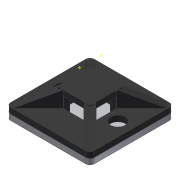
# Autodesk Inventor part: Klebesockel_HC-101SBK
Saved by Autodesk Inventor 2015 (Build 190159000, 159)
## iProperties
Created: 2015-01-25
Part Number: Klebesockel_HC-101SBK
Material: Generic
Document SubType Name: Modeling
Density: 1 g/cm^3
Appearance: Plastic_Black
Autodesk Inventor part; units mm, degrees
ref_plane "YZ Plane" through (0, 0, 0) normal (1, 0, 0) x (0, 1, 0)
sketch "Sketch1" plane through (0, 0, 0) normal (0, 0, 1) x (1, 0, 0)
  line L0 (-9.75, -9.75) -> (9.75, -9.75)
  line L1 (9.75, -9.75) -> (9.75, 9.75)
  line L2 (9.75, 9.75) -> (-9.75, 9.75)
  line L3 (-9.75, 9.75) -> (-9.75, -9.75)
  line L4 (-9.75, -9.75) -> (9.75, 9.75) construction
  line L5 (9.75, -9.75) -> (-9.75, 9.75) construction
  point P0 (0, 0)
  dimension "d0" = 19.5
  dimension "d1" = 19.5
  constraints: 12 end point, 2 midpoint, 2 parallel, 1 horizontal, 1 perpendicular
  measures "d0" distance of L2.end L1.end
  measures "d1" distance of L0.end L1.end
extrude "Extrusion1" add sketch "Sketch1" along normal blind 1.35
sketch "Sketch2" plane through (0, 0, 1.35) normal (0, 0, 1) x (1, 0, 0)
  line L0 (-3.8, -3.8) -> (3.8, -3.8)
  line L1 (3.8, -3.8) -> (3.8, 3.8)
  line L2 (3.8, 3.8) -> (-3.8, 3.8)
  line L3 (-3.8, 3.8) -> (-3.8, -3.8)
  line L4 (-3.8, -3.8) -> (3.8, 3.8) construction
  line L5 (3.8, -3.8) -> (-3.8, 3.8) construction
  point P0 (0, 0)
  dimension "d4" = 7.6
  dimension "d5" = 7.6
  constraints: 12 end point, 2 midpoint, 2 parallel, 1 horizontal, 1 perpendicular
  measures "d4" distance of L2.end L1.end
  measures "d5" distance of L0.end L1.end
extrude "Extrusion2" add sketch "Sketch2" along normal blind 3.7
fillet "Fillet1" radius 1 4 edges at (9.75, -9.75, 0.675) (9.75, 9.75, 0.675) (-9.75, -9.75, 0.675) (-9.75, 9.75, 0.675)
ref_plane "Work Plane1" through (0, 0, 0) normal (-0.7071, 0.7071, 0) x (0, 0, 1)
sketch "Sketch3" plane through (0, 0, 0) normal (-0.7071, 0.7071, 0) x (0, 0, 1)
  line L0 (5.05, 4.4) -> (1.35, 12.7)
  line L1 (1.35, 12.7) -> (1.35, 4.4)
  line L2 (1.35, 4.4) -> (5.05, 4.4)
  line L3 (1.35, 13.0815) -> (1.35, 0.7071) projected
  line L4 (5.05, 5.374) -> (5.05, 0) projected
  point P0 (0, 0)
  dimension "d10" = 4.4
  dimension "d11" = 12.7
  constraints: 6 end point, 1 collinear, 1 horizontal, 1 point on line, 1 vertical
  measures "d10" distance from line of point (0, 0) L2
  measures "d11" vertical distance of point (0, 0) L0.end
extrude "Extrusion3" add sketch "Sketch3" along normal mid plane 1.9
pattern_circular "Circular Pattern1" count 4 over 360 about axis through (0, 0, -10) along (0, 0, 1) of "Extrusion3"
sketch "Sketch4" plane through (0, 0, 0) normal (0, 0, -1) x (-1, 0, 0)
  line L0 (2.35, 3.8) -> (-2.35, 3.8)
  line L1 (-2.35, 3.8) -> (-2.35, -3.8)
  line L2 (-2.35, -3.8) -> (2.35, -3.8)
  line L3 (2.35, -3.8) -> (2.35, 3.8)
  line L4 (2.35, 3.8) -> (-2.35, -3.8) construction
  line L5 (-2.35, 3.8) -> (2.35, -3.8) construction
  line L6 (3.8, 2.35) -> (-3.8, 2.35)
  line L7 (-3.8, 2.35) -> (-3.8, -2.35)
  line L8 (-3.8, -2.35) -> (3.8, -2.35)
  line L9 (3.8, -2.35) -> (3.8, 2.35)
  line L10 (3.8, 2.35) -> (-3.8, -2.35) construction
  line L11 (-3.8, 2.35) -> (3.8, -2.35) construction
  line L12 (3.8, -3.8) -> (-3.8, -3.8) projected
  line L13 (-3.8, -3.8) -> (-3.8, 3.8) projected
  point P0 (0, 0)
  dimension "d17" = 4.7
  dimension "d18" = 4.7
  constraints: 24 end point, 4 midpoint, 4 parallel, 2 collinear, 2 horizontal, 2 perpendicular
  measures "d17" distance of L6.end L7.end
  measures "d18" distance of L1.end L2.end
extrude "Extrusion4" cut sketch "Sketch4" against normal blind 3.75 contours L3 L6 L1 L0 | L6 L9 L8 L3 | L3 L8 L1 L6 | L1 L8 L7 L6 | L3 L2 L1 L8
sketch "Sketch5" plane through (0, 0, 1.35) normal (0, 0, 1) x (1, 0, 0)
  point P0 (0, 0)
  point P1 (-6.5, 0)
  point P2 (6.5, 0)
  dimension "d22" = 13
  dimension "d23" = 6.5
  constraints: 2 horizontal alignment
  measures "d22" distance of point (6.5, 0) point (-6.5, 0)
  measures "d23" distance of point (0, 0) point (-6.5, 0)
hole "Hole1" at (-6.5, 0, 1.35) at (6.5, 0, 1.35) direction (0, 0, -1) diameter 3.4 end through all
sketch "Sketch6" plane through (0, 0, 0) normal (0, 0, -1) x (-1, 0, 0)
  line L0 (-8.75, 9.75) -> (8.75, 9.75) projected
  line L1 (-9.75, -8.75) -> (-9.75, 8.75) projected
  line L2 (8.75, -9.75) -> (-8.75, -9.75) projected
  line L3 (9.75, 8.75) -> (9.75, -8.75) projected
  arc A0 (8.75, -9.75) -> (9.75, -8.75) centre (8.75, -8.75) ccw projected
  arc A1 (-9.75, -8.75) -> (-8.75, -9.75) centre (-8.75, -8.75) ccw projected
  arc A2 (-8.75, 9.75) -> (-9.75, 8.75) centre (-8.75, 8.75) ccw projected
  arc A3 (9.75, 8.75) -> (8.75, 9.75) centre (8.75, 8.75) ccw projected
extrude "Extrusion5" add sketch "Sketch6" along normal blind 1.3 separate body
ref_plane "Work Plane2" through (0, 0, 10.05) normal (0, 0, 1) x (1, 0, 0)
sketch "Sketch7" plane through (0, 0, 10.05) normal (0, 0, 1) x (1, 0, 0)
  point P0 (0, 0)
  point P1 (0, -2.5)
  point P2 (0, 2.5)
  dimension "d34" = 5
  dimension "d35" = 2.5
  constraints: 2 vertical alignment
  measures "d34" distance of point (0, 2.5) point (0, -2.5)
  measures "d35" distance of point (0, 0) point (0, -2.5)
equation "\"d1\" = d0"
equation "\"d5\" = d4"
equation "\"d18\" = d17"
equation "\"d23\" = 0.5 * d22"
equation "\"d35\" = 0.5 * d34"
body "Solid1"
body "Solid2"
